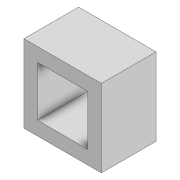
# Autodesk Inventor part: Base
Saved by Autodesk Inventor 2020 (Build 240168000, 168)
## iProperties
Created: 2021-05-19
Part Number: Base
Material: Generic
Document SubType Name: Modeling
Designer: deox
Density: 1 g/cm^3
Appearance: Default
Author: deox
Autodesk Inventor part; units mm, degrees
ref_plane "YZ Plane" through (0, 0, 0) normal (1, 0, 0) x (0, 1, 0)
ref_plane "XZ Plane" through (0, 0, 0) normal (0, 1, 0) x (-1, 0, 0)
ref_plane "XY Plane" through (0, 0, 0) normal (0, 0, 1) x (1, 0, 0)
sketch "Sketch1" plane through (0, 0, 0) normal (0, 0, 1) x (1, 0, 0)
  line L0 (-2.75, -2.75) -> (2.75, -2.75)
  line L1 (2.75, -2.75) -> (2.75, 2.75)
  line L2 (2.75, 2.75) -> (-2.75, 2.75)
  line L3 (-2.75, 2.75) -> (-2.75, -2.75)
  line L4 (-2.75, -2.75) -> (2.75, 2.75) construction
  line L5 (2.75, -2.75) -> (-2.75, 2.75) construction
  line L6 (-4.25, -4.25) -> (4.25, -4.25)
  line L7 (4.25, -4.25) -> (4.25, 4.25)
  line L8 (4.25, 4.25) -> (-4.25, 4.25)
  line L9 (-4.25, 4.25) -> (-4.25, -4.25)
  line L10 (-4.25, -4.25) -> (4.25, 4.25) construction
  line L11 (4.25, -4.25) -> (-4.25, 4.25) construction
  point P0 (0, 0)
  dimension "d0" = 5.5
  dimension "d1" = 5.5
  dimension "d2" = 8.5
  dimension "d3" = 8.5
  constraints: 24 end point, 4 midpoint, 4 parallel, 2 horizontal, 2 perpendicular
  measures "d0" distance of L2.end L1.end
  measures "d1" distance of L1.end L0.end
  measures "d2" distance of L8.end L7.end
  measures "d3" distance of L7.end L6.end
extrude "Extrusion1" add sketch "Sketch1" along normal blind 6
body "Solid1"
